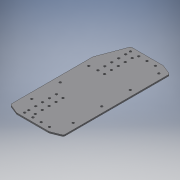
# Autodesk Inventor part: 足裏_アングル
Saved by Autodesk Inventor 2018 (Build 220112000, 112)
## iProperties
Created: 2016-05-13
Part Number: 足裏_アングル
Material: GFRP
Document SubType Name: Modeling
Designer: hiroaki
Density: 1.75 g/cm^3
Appearance: 滑らか - 淡い灰色
Mass: 33.025 g
Surface Area: 212.008 cm^2
Volume: 18.8714 cm^3
Author: hiroaki
Autodesk Inventor part; units mm, degrees
ref_plane "YZ Plane" through (0, 0, 0) normal (1, 0, 0) x (0, 1, 0)
ref_plane "XZ Plane" through (0, 0, 0) normal (0, 1, 0) x (-1, 0, 0)
ref_plane "XY Plane" through (0, 0, 0) normal (0, 0, 1) x (1, 0, 0)
sketch "スケッチ1" plane through (0, 0, 0) normal (0, 0, 1) x (1, 0, 0)
  circle A0 centre (-4.75, 50) radius 1.55
  circle A1 centre (4.75, 50) radius 1.55
  circle A2 centre (-4.75, -50) radius 1.55
  circle A3 centre (4.75, -50) radius 1.55
  line L0 (-4.75, -50) -> (4.75, -50) construction
  line L1 (4.75, -50) -> (4.75, 50) construction
  line L2 (4.75, 50) -> (-4.75, 50) construction
  line L3 (-4.75, 50) -> (-4.75, -50) construction
  line L4 (-4.75, -50) -> (4.75, 50) construction
  line L5 (4.75, -50) -> (-4.75, 50) construction
  circle A4 centre (19.25, 57) radius 1.55
  circle A5 centre (31.25, 57) radius 1.55
  circle A6 centre (19.25, -96) radius 1.55
  circle A7 centre (31.25, -96) radius 1.55
  circle A8 centre (7.25, 57) radius 1.55
  circle A9 centre (-4.75, 57) radius 1.55
  circle A10 centre (7.25, -96) radius 1.55
  circle A11 centre (-4.75, -96) radius 1.55
  circle A12 centre (4.75, 50) radius 2.75 construction
  circle A13 centre (-4.75, 40) radius 1.55
  circle A14 centre (4.75, 40) radius 1.55
  circle A15 centre (-4.75, -60) radius 1.55
  circle A16 centre (4.75, -60) radius 1.55
  circle A17 centre (-4.75, 30) radius 1.55
  circle A18 centre (4.75, 30) radius 1.55
  circle A19 centre (-4.75, -70) radius 1.55
  circle A20 centre (4.75, -70) radius 1.55
  circle A21 centre (-4.75, 20) radius 1.55
  circle A22 centre (4.75, 20) radius 1.55
  circle A23 centre (-4.75, -80) radius 1.55
  circle A24 centre (4.75, -80) radius 1.55
  circle A25 centre (-4.75, 10) radius 1.55
  circle A26 centre (4.75, 10) radius 1.55
  circle A27 centre (-4.75, -90) radius 1.55
  circle A28 centre (4.75, -90) radius 1.55
  line L6 (-25.25, 23) -> (-10.25, 63)
  line L7 (51.75, 57) -> (36.75, 63)
  line L8 (36.75, -102) -> (51.75, -96)
  line L9 (-10.25, -102) -> (-25.25, -96)
  line L10 (-10.25, 63) -> (36.75, 63)
  line L11 (51.75, 57) -> (51.75, -96)
  line L12 (36.75, -102) -> (-10.25, -102)
  line L13 (-25.25, -96) -> (-25.25, 23)
  circle A29 centre (43.25, 50) radius 1.55
  circle A30 centre (43.25, 8.75) radius 1.55
  circle A31 centre (43.25, -32.5) radius 1.55
  circle A32 centre (43.25, -73.75) radius 1.55
  circle A33 centre (-16.75, -73.75) radius 1.55
  circle A34 centre (-16.75, -32.5) radius 1.55
  circle A35 centre (-16.75, 8.75) radius 1.55
  line L14 (-4.75, -96) -> (31.25, -96) construction
  line L15 (-4.75, 57) -> (31.25, 57) construction
  line L16 (13.25, -99.8993) -> (13.25, -85.1229) construction
  line L17 (13.25, 59.3052) -> (13.25, 46.6028) construction
  point P0 (0, 0)
  point P1 (0, 0)
  point P2 (0, 0)
  dimension "d0" = 3.1
  dimension "d1" = 9.5
  dimension "d2" = 100
  dimension "d41" = 5.5
  dimension "d47" = 10
  dimension "d54" = 77
  dimension "d55" = 165
  dimension "d56" = 3.1
  dimension "d59" = 41.25
  dimension "d64" = 3.1
  dimension "d67" = 41.25
  dimension "d75" = 15
  dimension "d76" = 15
  dimension "d77" = 15
  dimension "d78" = 15
  dimension "d79" = 20.5
  dimension "d80" = 52
  dimension "d81" = 8.5
  dimension "d82" = 28.25
  dimension "d83" = 8.5
  dimension "d84" = 13
  dimension "d85" = 6
  dimension "d87" = 12
  dimension "d88" = 12
  dimension "d89" = 12
  dimension "d90" = 6
  dimension "d91" = 12
  dimension "d92" = 12
  dimension "d94" = 12
  dimension "d95" = 6
  dimension "d96" = 6
  dimension "d97" = 6
  dimension "d98" = 40
  constraints: 36 centre point, 36 end point, 11 coincident, 11 equal radius, 6 vertical, 4 point on line, 3 horizontal, 3 midpoint, 2 parallel, 2 symmetric about line, 49 other
  measures "d0" diameter of A1
  measures "d1" distance of L1.end L2.end
  measures "d2" distance of L0.end L1.end
  measures "d41" diameter of A12
  measures "d47" distance of A0.centre A13.centre
  measures "d54" distance between parallel lines of L13 L11
  measures "d55" distance between parallel lines of L10 L12
  measures "d56" diameter of A29
  measures "d59" distance of A29.centre A30.centre
  measures "d64" diameter of A33
  measures "d67" distance of A33.centre A34.centre
  measures "d75" distance from line of L9.start L13
  measures "d76" distance from line of L11 L8.start
  measures "d77" horizontal distance of L6.end L6.start
  measures "d78" horizontal distance of L7.start L7.end
  measures "d79" distance between parallel lines of L3 L13
  measures "d80" distance between parallel lines of L12 L0
  measures "d81" distance from line of L13 A33.centre
  measures "d82" distance from line of L12 point (-16.75, -73.75)
  measures "d83" distance from line of L11 A29.centre
  measures "d84" distance from line of L10 A29.centre
  measures "d85" distance from line of L12 L14.start
  measures "d87" distance of A10.centre L14.start
  measures "d88" distance of A6.centre A10.centre
  measures "d89" distance of L14.end A6.centre
  measures "d90" distance between parallel lines of L10 L15
  measures "d91" distance of A8.centre L15.start
  measures "d92" distance of A4.centre A8.centre
  measures "d94" distance of L15.end A4.centre
  measures "d95" distance from line of L9.end L12
  measures "d96" distance from line of L8.end L12
  measures "d97" distance from line of L7.start L10
  measures "d98" vertical distance of L6.start L6.end
extrude "押し出し4" add sketch "スケッチ1" along normal blind 2
fillet "フィレット2" radius 3 8 edges at (-10.25, -102, 1) (-25.25, -96, 1) (36.75, -102, 1) (51.75, -96, 1) (-25.25, 23, 1) (-10.25, 63, 1) (36.75, 63, 1) (51.75, 57, 1)
equation "\"d1\" = d20"
equation "\"H_head\" = 28.5"
equation "\"H_leg\" = 199.5"
equation "\"足の面積\" = 12720.125"
equation "\"現在の面積\" = 11560"
equation "\"足_短辺\" = 68"
equation "\"円柱\" = 313.5"
equation "\"胴体中心から手先\" = 342"
equation "\"H_leg_1\" = 186.2"
equation "\"H_leg_MAX\" = 399"
equation "\"H_head_1\" = 26.6"
equation "\"H_head_MAX\" = 142.5"
equation "\"d20\" = 9.5"
